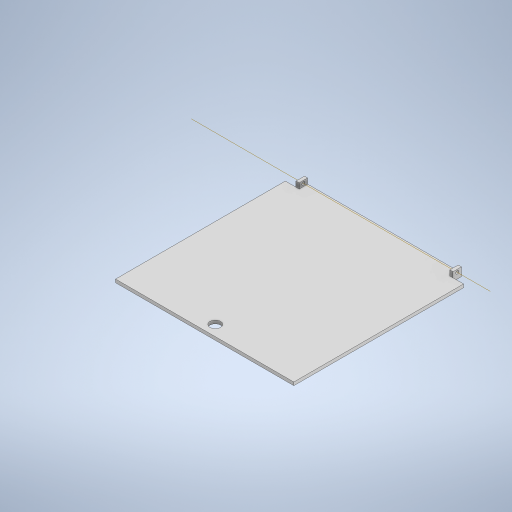
# Autodesk Inventor part: Cabinet - door
Saved by Autodesk Inventor 2024.3 (Build 283343000, 343)
## iProperties
Created: 2025-03-26
Part Number: Cabinet - door
Material: Všeobecné
Document SubType Name: Modeling
Designer: admin
Density: 1 g/cm^3
Appearance: Výchozí
Author: admin
Autodesk Inventor part; units mm, degrees
ref_plane "YZ Plane" through (0, 0, 0) normal (1, 0, 0) x (0, 1, 0)
ref_plane "XZ Plane" through (0, 0, 0) normal (0, 1, 0) x (-1, 0, 0)
ref_plane "XY Plane" through (0, 0, 0) normal (0, 0, 1) x (1, 0, 0)
sketch "Náčrt1" plane through (0, 0, 0) normal (0, 1, 0) x (-1, 0, 0)
  line L0 (84, 84) -> (-84, 84)
  line L1 (-84, 84) -> (-84, -84)
  line L2 (-84, -84) -> (84, -84)
  line L3 (84, -84) -> (84, 84)
  line L4 (0, -117.6) -> (0, 117.6) projected
  line L5 (-117.6, 0) -> (117.6, 0) projected
  point P0 (0, 0)
  dimension "d0" = 168
  dimension "d1" = 168
  constraints: 8 end point, 2 parallel, 1 horizontal, 1 perpendicular, 2 other
  measures "d0" distance of L0.end L1.end
  measures "d1" distance of L0.start L0.end
extrude "Vysunutí1" add sketch "Náčrt1" along normal mid plane 3
sketch "Náčrt2" plane through (0, 1.5, 0) normal (0, 1, 0) x (1, 0, 0)
  line L0 (-84, -84) -> (84, -84) projected
  line L1 (84, -84) -> (84, 84) projected
  point P0 (0, 0)
  point P1 (0, -74)
  dimension "d13" = 10
  dimension "d14" = 84
  measures "d13" distance from line of L0 point (0, -74)
  measures "d14" distance from line of L1 point (0, -74)
sketch "Náčrt3" plane through (0, 1.5, 0) normal (0, 1, 0) x (1, 0, 0)
  line L0 (74, 84) -> (84, 84)
  line L1 (84, 84) -> (84, 76)
  line L2 (84, 76) -> (74, 76)
  line L3 (74, 76) -> (74, 84)
  line L4 (84, 84) -> (-84, 84) projected
  line L5 (84, -84) -> (84, 84) projected
  point P0 (0, 0)
  dimension "d9" = 10
  dimension "d10" = 8
  constraints: 8 end point, 2 collinear, 2 parallel, 1 horizontal, 1 perpendicular
  measures "d9" distance of L1.end L2.end
  measures "d10" distance of L2.end L0.start
extrude "Vysunutí3" cut sketch "Náčrt3" against normal through all
mirror "Zrcadlit1" about plane through (0, 0, 0) normal (1, 0, 0) of "Vysunutí3"
hole "Díra1" at (0, 1.5, 74) direction (0, -1, 0) diameter 10 end through all
sketch "Náčrt4" plane through (0, 1.5, 0) normal (0, 1, 0) x (1, 0, 0)
  line L0 (71, 76) -> (74, 76)
  line L1 (74, 76) -> (74, 84)
  line L2 (74, 84) -> (71, 84)
  line L3 (71, 84) -> (71, 76)
  line L4 (74, 76) -> (74, 84) projected
  line L5 (74, 84) -> (-74, 84) projected
  point P0 (0, 0)
  dimension "d22" = 3
  constraints: 8 end point, 3 collinear, 2 parallel, 1 horizontal, 1 perpendicular
  measures "d22" distance of L0.start L0.end
extrude "Vysunutí4" add sketch "Náčrt4" along normal blind 5
sketch "Náčrt5" plane through (74, -1.5, -76) normal (1, 0, 0) x (0, 0, -1)
  line L0 (0, 8) -> (8, 8) projected
  line L1 (0, 3) -> (0, 8) projected
  line L2 (8, 8) -> (8, 0) projected
  point P0 (-76, 1.5)
  point P1 (4, 5.5)
  dimension "d25" = 2.5
  dimension "d34" = 4
  measures "d25" distance from line of L0 point (4, 5.5)
  measures "d34" distance from line of L2 point (4, 5.5)
hole "Díra2" at (74, 4, -80) direction (-1, 0, 0) diameter 3 depth 3
mirror "Zrcadlit2" about plane through (0, 0, 0) normal (1, 0, 0) of "Vysunutí4", "Díra2"
